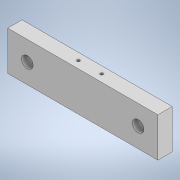
# Autodesk Inventor part: Endschalterhalter
Saved by Autodesk Inventor 2021 (Build 250183000, 183)
## iProperties
Created: 2024-06-30
Part Number: Endschalterhalter
Material: Generic
Document SubType Name: Modeling
Designer: Lukas
Density: 1 g/cm^3
Appearance: Default
Author: Lukas
Autodesk Inventor part; units mm, degrees
ref_plane "YZ Plane" through (0, 0, 0) normal (1, 0, 0) x (0, 1, 0)
ref_plane "XZ Plane" through (0, 0, 0) normal (0, 1, 0) x (-1, 0, 0)
ref_plane "XY Plane" through (0, 0, 0) normal (0, 0, 1) x (1, 0, 0)
sketch "Sketch1" plane through (0, 0, 0) normal (0, 0, 1) x (1, 0, 0)
  line L0 (-21, 5.5) -> (21, 5.5)
  line L1 (21, 5.5) -> (21, -5.5)
  line L2 (21, -5.5) -> (-21, -5.5)
  line L3 (-21, -5.5) -> (-21, 5.5)
  circle A0 centre (-15.5, 0) radius 1.6
  circle A1 centre (15.5, 0) radius 1.6
  point P0 (0, 0)
  point P1 (0, 5.5)
  point P2 (-21, 0)
  dimension "d0" = 31
  dimension "d1" = 15.5
  dimension "d2" = 5.5
  dimension "d3" = 5.5
  dimension "d4" = 3.2
  constraints: 8 end point, 3 horizontal alignment, 2 centre point, 2 midpoint, 2 parallel, 1 equal radius, 1 horizontal, 1 perpendicular, 1 vertical alignment
  measures "d0" distance of A1.centre A0.centre
  measures "d1" distance of point (0, 0) A0.centre
  measures "d2" distance from line of L0 A0.centre
  measures "d3" distance from line of L3 A0.centre
  measures "d4" diameter of A0
extrude "Extrusion1" add sketch "Sketch1" along normal blind 4
sketch "Sketch2" plane through (-21, 5.5, 0) normal (0, 1, 0) x (1, 0, 0)
  circle A0 centre (24.25, -2) radius 0.4
  circle A1 centre (17.75, -2) radius 0.4
  line L0 (0, 0) -> (0, -4) projected
  point P0 (21, 0)
  point P1 (0, -2)
  dimension "d7" = 6.5
  dimension "d8" = 3.25
  dimension "d9" = 0.8
  constraints: 2 centre point, 2 horizontal alignment, 1 equal radius, 1 midpoint
  measures "d7" distance of A0.centre A1.centre
  measures "d8" horizontal distance of point (21, 0) A1.centre
  measures "d9" diameter of A0
extrude "Extrusion2" cut sketch "Sketch2" against normal through all
equation "\"d1\" = 0.5 * d0"
equation "\"d8\" = 0.5 * d7"
body "Solid1"
